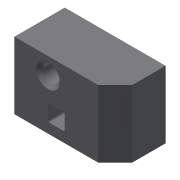
# Autodesk Inventor part: pc01
Saved by Autodesk Inventor 2022 Beta2 (Build 260130000, 130) ContinuousBuild 0
## iProperties
Shininess: 64.0
Length Units: 11269
Angle Units: 11279
Time Units: 11290
Mass Units: 11283
Length Display Precision: 3
Angle Display Precision: 2
Compacted: True
Part Number: pc01
Document SubType Name: Modeling
Created: 2004-04-15
Designer: mpaknia
Manufacturer: Standard
Standards Organization: Custom
Density: 1 g/cm^3
Material: Generic
Appearance: Light Gray
Density: 0.0
Volumn: 0.0
Area: 0.0
PropertySet Name: Model Information
Control State: 0
Master: False
Checked Out: False
Author: mpaknia
Autodesk Inventor part; units mm, degrees
ref_plane "YZ Plane" through (0, 0, 0) normal (1, 0, 0) x (0, 1, 0)
ref_plane "XZ Plane" through (0, 0, 0) normal (0, 1, 0) x (-1, 0, 0)
ref_plane "XY Plane" through (0, 0, 0) normal (0, 0, 1) x (1, 0, 0)
sketch "Sketch1" plane through (0, 0, 0) normal (0, 0, 1) x (1, 0, 0)
  line L0 (0, 0) -> (150, 0)
  line L1 (150, 0) -> (150, 75)
  line L2 (150, 75) -> (0, 75)
  line L3 (0, 75) -> (0, 0)
  dimension "d0" = 150
  dimension "d1" = 75
  constraints: 8 end point, 2 parallel, 1 horizontal, 1 perpendicular
  measures "d0" distance between parallel lines of L1 L3
  measures "d1" distance between parallel lines of L0 L2
extrude "Extrusion1" add sketch "Sketch1" along normal blind 100
chamfer "Chamfer1" distance 25 angle 45 1 edges at (150, 0, 50)
sketch "Sketch2" plane through (0, 0, 0) normal (0, -1, 0) x (1, 0, 0)
  line L0 (125, 100) -> (0, 100) projected
  line L1 (0, 0) -> (0, 100) projected
  point P0 (50, 75)
  dimension "d7" = 25
  dimension "d8" = 50
  measures "d7" distance from line of L0 point (50, 75)
  measures "d8" distance from line of L1 point (50, 75)
hole "Hole1" at (50, 0, 75) direction (0, 1, 0) diameter 25 end through all
sketch "Sketch3" plane through (0, 0, 0) normal (0, -1, 0) x (1, 0, 0)
  line L0 (75, 40) -> (50, 40)
  line L1 (50, 40) -> (50, 15)
  line L2 (50, 15) -> (75, 15)
  line L3 (75, 15) -> (75, 40)
  line L4 (125, 100) -> (125, 0) projected
  circle A0 centre (50, 75) radius 12.5 projected
  dimension "d16" = 25
  dimension "d17" = 50
  dimension "d18" = 35
  constraints: 8 end point, 2 parallel, 2 perpendicular, 1 horizontal
  measures "d16" distance of L0.start L0.end
  measures "d17" distance between parallel lines of L4 L3
  measures "d18" distance from line of A0.centre L0
extrude "Extrusion2" cut sketch "Sketch3" against normal through all contours L3 L2 L1 L0
fillet "Fillet1" radius 3 4 edges at (50, 37.5, 15) (75, 37.5, 15) (50, 37.5, 40) (75, 37.5, 40)
chamfer "Chamfer2" distance 5 angle 45 1 edges at (50, 0, 87.5)
body "Solid1"
